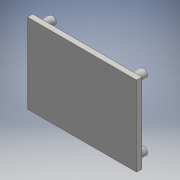
# Autodesk Inventor part: TrolleyTopPlate1
Saved by Autodesk Inventor 2016 (Build 200138000, 138)
## iProperties
Created: 2016-03-28
Part Number: TrolleyTopPlate1
Material: Generic
Document SubType Name: Modeling
Designer: mkepler
Density: 1 g/cm^3
Appearance: Default
Mass: 8.67871 g
Surface Area: 68.4002 cm^2
Volume: 8.67871 cm^3
Author: mkepler
Autodesk Inventor part; units mm, degrees
ref_plane "YZ Plane" through (0, 0, 0) normal (1, 0, 0) x (0, 1, 0)
ref_plane "XZ Plane" through (0, 0, 0) normal (0, 1, 0) x (-1, 0, 0)
ref_plane "XY Plane" through (0, 0, 0) normal (0, 0, 1) x (1, 0, 0)
sketch "Sketch1" plane through (0, 0, 0) normal (0, 1, 0) x (-1, 0, 0)
  line L0 (0, 0) -> (61.5, 0)
  line L1 (61.5, 0) -> (61.5, -45)
  line L2 (61.5, -45) -> (0, -45)
  line L3 (0, -45) -> (0, 0)
  dimension "d0" = 61.5
  dimension "d1" = 45
  constraints: 8 end point, 2 parallel, 1 horizontal, 1 perpendicular
  measures "d0" distance of L1.end L2.end
  measures "d1" distance of L0.end L1.end
extrude "Extrusion1" add sketch "Sketch1" along normal blind 3
sketch "Sketch2" plane through (0, 3, 0) normal (0, 1, 0) x (1, 0, 0)
  circle A0 centre (-27, 25.5) radius 2.5
  line L0 (0, 0) -> (0, 45) projected
  line L1 (-61.5, 0) -> (0, 0) projected
  line L2 (0, 45) -> (-61.5, 45) projected
  circle A1 centre (-39, 25.4996) radius 2.5
  circle A2 centre (-38.887, 7.5) radius 2.5
  circle A3 centre (-27, 7.5) radius 2.5
  dimension "d4" = 5
  dimension "d5" = 27
  dimension "d8" = 5
  dimension "d9" = 12
  dimension "d10" = 5
  dimension "d11" = 18
  dimension "d12" = 5
  dimension "d13" = 7.5
  dimension "d14" = 7.5
  dimension "d15" = 18
  constraints: 4 centre point
  measures "d4" diameter of A0
  measures "d5" distance from line of L0 A0.centre
  measures "d8" diameter of A1
  measures "d9" distance of A1.centre A0.centre
  measures "d10" diameter of A2
  measures "d11" distance of A1.centre A2.centre
  measures "d12" diameter of A3
  measures "d13" distance from line of L1 A2.centre
  measures "d14" distance from line of L1 A3.centre
  measures "d15" distance of A3.centre A0.centre
hole "Hole1" at (-27, 3, -7.5) at (-38.887, 3, -7.5) at (-39, 3, -25.4996) at (-27, 3, -25.5) direction (0, -1, 0) diameter 5 depth 2.5
sketch "Sketch3" plane through (0, 3, 0) normal (0, 1, 0) x (1, 0, 0)
  circle A0 centre (-5, 3.5) radius 2.25
  line L0 (-61.5, 0) -> (0, 0) projected
  line L1 (0, 0) -> (0, 45) projected
  circle A1 centre (-56.5, 3.5) radius 2.25
  line L2 (-61.5, 45) -> (-61.5, 0) projected
  circle A2 centre (-5, 41.5) radius 2.25
  line L3 (0, 45) -> (-61.5, 45) projected
  circle A3 centre (-56.5, 41.5) radius 2.25
  circle A4 centre (-29.5, 41.5) radius 2.25
  circle A5 centre (-36.5, 41.5) radius 2.25
  dimension "d23" = 4.5
  dimension "d24" = 3.5
  dimension "d25" = 5
  dimension "d26" = 4.5
  dimension "d27" = 3.5
  dimension "d28" = 5
  dimension "d29" = 4.5
  dimension "d30" = 3.5
  dimension "d31" = 4.5
  dimension "d32" = 4.5
  dimension "d33" = 24.5
  dimension "d34" = 5
  dimension "d35" = 5
  dimension "d36" = 3.5
  dimension "d37" = 4.5
  dimension "d38" = 20
  constraints: 6 centre point
  measures "d23" diameter of A0
  measures "d24" distance from line of L0 A0.centre
  measures "d25" distance from line of L1 A0.centre
  measures "d26" diameter of A1
  measures "d27" distance from line of L0 A1.centre
  measures "d28" distance from line of A1.centre L2
  measures "d29" diameter of A2
  measures "d30" distance from line of L3 A2.centre
  measures "d31" diameter of A3
  measures "d32" diameter of A4
  measures "d33" distance of A4.centre A2.centre
  measures "d34" distance from line of L2 A3.centre
  measures "d35" distance from line of L1 A2.centre
  measures "d36" distance from line of L3 A3.centre
  measures "d37" diameter of A5
  measures "d38" distance of A3.centre A5.centre
extrude "Extrusion2" add sketch "Sketch3" along normal blind 6 contours A0 | A1 | A2 | A3 | A4 | A5
body "Solid1"
